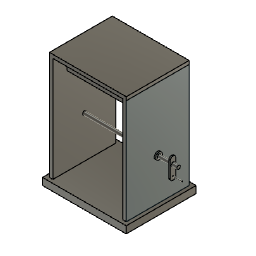
Butterfly Automata Toy v2 (Autodesk Fusion 360 design; units mm, degrees)
Autodesk Fusion 360 part; units mm, degrees
sketch "Box" plane through (0, 0, 0) normal (0, 0, 1) x (1, 0, 0) in component "Box"
  line L0 (0, 50) -> (60, 50)
  line L1 (60, 50) -> (60, 0)
  line L2 (-60, 50) -> (-60, 0)
  line L3 (0, 50) -> (-60, 50)
  line L4 (60, -50) -> (60, 0)
  line L5 (0, -50) -> (60, -50)
  line L6 (0, -50) -> (-60, -50)
  line L7 (-60, -50) -> (-60, 0)
  line L8 (-55, 45) -> (-49.9845, 45)
  line L9 (-49.9845, 45) -> (-49.9845, -45)
  line L10 (-49.9845, -45) -> (-55, -45)
  line L11 (-55, -45) -> (-55, 45)
  line L12 (0, 50) -> (0, -50)
  line L13 (49.9845, 45) -> (49.9845, -45)
  line L14 (55, 45) -> (49.9845, 45)
  line L15 (55, -45) -> (55, 45)
  line L16 (49.9845, -45) -> (55, -45)
  dimension "d1" = 60
  dimension "d5" = 90
  constraint horizontal L0
  constraint vertical L1
  constraint horizontal L8
  constraint vertical L9
  constraint horizontal L10
  constraint vertical L11
  constraint perpendicular L6 L12
  constraint symmetric L8.start L12 L14.start
  constraint symmetric L8.end L12 L13.start
  constraint symmetric L9.end L12 L13.end
  constraint symmetric L10.end L12 L15.start
  measures "d1" distance of L0.start L0.end
  measures "d5" distance of L8.start L10.end
extrude "Extrude1" add sketch "Box" along normal blind 10 contours L2 L3 L6 L7 L12 | L0 L1 L4 L5 L12 | L8 L9 L10 L11 | L13 L14 L15 L16 makes body 1 in component "Box"
extrude "Extrude2" add sketch "Box" along normal blind 160 contours L8 L9 L10 L11 | L13 L14 L15 L16 bodies 1 in component "Box"
sketch "Cover" plane through (-49.9845, 0, 0) normal (1, 0, 0) x (0, 1, 0) in component "Box"
  line L0 (-45, 10) -> (45, 10)
  line L1 (45, 10) -> (45, 160)
  line L2 (45, 160) -> (-45, 160)
  line L3 (-45, 160) -> (-45, 10)
  line L4 (0, 140) -> (25, 140)
  line L5 (25, 140) -> (25, 135)
  line L6 (25, 135) -> (0, 135)
  line L7 (0, 140) -> (-25, 140)
  line L8 (-25, 140) -> (-25, 135)
  line L9 (-25, 135) -> (0, 135)
  line L10 (45, 160) -> (-45, 160)
  line L11 (-45, 160) -> (-45, 165)
  line L12 (-45, 165) -> (45, 165)
  line L13 (45, 165) -> (45, 160)
  circle A0 centre (0, 70) radius 2.5
  dimension "d8" = 25
  dimension "d9" = 5
  dimension "d12" = 90
  dimension "d13" = 5
  dimension "d18" = 5
  constraint horizontal L4
  constraint vertical L5
  constraint horizontal L6
  constraint horizontal L10
  constraint vertical L11
  constraint horizontal L12
  constraint vertical L13
  constraint coincident L1.end L2.start
  measures "d8" distance of L4.start L4.end
  measures "d9" distance of L4.start L6.end
  measures "d12" distance of L1.end L2.end
  measures "d13" distance of L1.end L12.end
  measures "d18" diameter of A0
extrude "Extrude3" add sketch "Cover" along normal blind 102 contours L4 L5 L6 L7 L8 L9 bodies 1 in component "Box"
extrude "Extrude4" add sketch "Cover" along normal blind 105 and the other way blind 5 contours L2 L10 L11 L12 L13 bodies 1 in component "Box"
extrude "Extrude5" cut sketch "Cover" along normal blind 150 and the other way blind 20 contours A0 bodies 1 in component "Box"
sketch "axe" plane through (55, 0, 0) normal (1, 0, 0) x (0, 1, 0) in component "Axe"
  circle A0 centre (0, 70) radius 2.5
  line L0 (-45, 10) -> (45, 10)
  line L1 (45, 10) -> (45, 160)
  line L2 (45, 160) -> (-45, 160)
  line L3 (-45, 160) -> (-45, 10)
  circle A1 centre (0, 70) radius 2.5
  circle A2 centre (0, 70) radius 5
  dimension "d23" = 5
  dimension "d24" = 10
  constraint concentric A0 A1
  constraint concentric A0 A2
  measures "d23" diameter of A1
  measures "d24" diameter of A2
extrude "Extrude1'" add sketch "axe" along normal blind 20 and the other way blind 120 separate body contours A0 A1 makes body 2 in component "Axe"
extrude "Extrude2'" add sketch "axe" along normal blind 2 contours A2 bodies 2 in component "Axe"
sketch "Sketch1" plane through (55, 0, 0) normal (1, 0, 0) x (0, 1, 0)
  circle A0 centre (0, 70) radius 2.5
  line L0 (-45, 10) -> (45, 10)
  line L1 (45, 10) -> (45, 160)
  line L2 (45, 160) -> (-45, 160)
  line L3 (-45, 160) -> (-45, 10)
sketch "handle" plane through (75, 0, 0) normal (1, 0, 0) x (0, 1, 0) in component "Handle"
  circle A0 centre (0, 70) radius 2.5
  line L0 (4, 70) -> (4, 76.5)
  line L1 (0.5, 80) -> (-0.5, 80)
  line L2 (-4, 76.5) -> (-4, 70)
  line L3 (-4, 70) -> (-4, 53.5)
  line L4 (-0.5, 50) -> (0.5, 50)
  line L5 (4, 53.5) -> (4, 70)
  circle A1 centre (0, 70) radius 2.5
  arc A2 (-0.5, 80) -> (-4, 76.5) centre (-0.5, 76.5) ccw
  arc A3 (4, 76.5) -> (0.5, 80) centre (0.5, 76.5) ccw
  arc A4 (0.5, 50) -> (4, 53.5) centre (0.5, 53.5) ccw
  arc A5 (-4, 53.5) -> (-0.5, 50) centre (-0.5, 53.5) ccw
  circle A6 centre (0, 55) radius 0.75
  point P0 (4, 50)
  dimension "d31" = 8
  dimension "d32" = 20
  dimension "d35" = 3.5
  dimension "d36" = 3.5
  dimension "d39" = 1.5
  constraint vertical L0
  constraint horizontal L1
  constraint vertical L2
  constraint vertical L3
  constraint horizontal L4
  constraint vertical L5
  constraint concentric A0 A1
  constraint tangent L1 A2
  constraint tangent L2 A2
  constraint tangent L0 A3
  constraint tangent L1 A3
  constraint equal A2 A3
  constraint coincident P0 L4
  constraint coincident P0 L5
  constraint tangent L4 A4
  constraint tangent L5 A4
  constraint tangent L3 A5
  constraint tangent L4 A5
  constraint equal A4 A5
  measures "d31" distance of L0.start L2.end
  measures "d32" distance of L0.start P0
  measures "d35" radius of A2
  measures "d36" radius of A4
  measures "d39" diameter of A6
extrude "Extrude3'" add 1 faces at (75, -1.687, 69.5683) along direction (1, 0, 0) blind 10 on bodies 2 bodies 2 in component "Axe"
extrude "Extrude1''" add sketch "handle" along normal blind 2 separate body contours L0 L1 L2 L3 L4 L5 A2 A3 A4 A5 | A6 makes body 3 in component "Handle"
extrude "Extrude2''" cut sketch "handle" along normal blind 5 contours A6 bodies 3 in component "Handle"
extrude "Extrude3''" add sketch "handle" along normal blind 15 and the other way blind 2 contours A6 bodies 3 in component "Handle"
component "Box" placed x (1, 0, 0) y (0, 1, 0) z (0, 0, 1) at (0, 0, 0)
component "Disks" placed x (1, 0, 0) y (0, 1, 0) z (0, 0, 1) at (0, 0, 0)
component "Axe" placed x (1, 0, 0) y (0, 1, 0) z (0, 0, 1) at (0, 0, 0)
component "Handle" placed x (1, 0, 0) y (0, 1, 0) z (0, 0, 1) at (0, 0, 0)
component "Connecting rods" placed x (1, 0, 0) y (0, 1, 0) z (0, 0, 1) at (0, 0, 0)
component "Butterfly" placed x (1, 0, 0) y (0, 1, 0) z (0, 0, 1) at (0, 0, 0)
component "Disk 1" placed x (1, 0, 0) y (0, 1, 0) z (0, 0, 1) at (0, 0, 0) in component "Disks"
component "Disk 2" placed x (1, 0, 0) y (0, 1, 0) z (0, 0, 1) at (0, 0, 0) in component "Disks"
component "Disk 3" placed x (1, 0, 0) y (0, 1, 0) z (0, 0, 1) at (0, 0, 0) in component "Disks"
component "Connecting rod 1" placed x (1, 0, 0) y (0, 1, 0) z (0, 0, 1) at (0, 0, 0) in component "Connecting rods"
component "Connecting rod 2" placed x (1, 0, 0) y (0, 1, 0) z (0, 0, 1) at (0, 0, 0) in component "Connecting rods"
component "Connecting rod 3" placed x (1, 0, 0) y (0, 1, 0) z (0, 0, 1) at (0, 0, 0) in component "Connecting rods"
